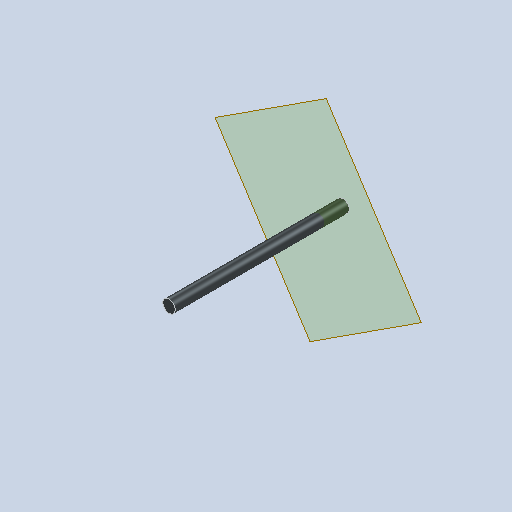
# Autodesk Inventor part: вал
Saved by Autodesk Inventor 2024.2 (Build 282272000, 272)
## iProperties
Created: 2025-11-23
Part Number: вал
Material: Типовые
Document SubType Name: Modeling
Designer: katya_notebook
Density: 1 g/cm^3
Appearance: Чугун серый
Mass: 1.37445 g
Surface Area: 11.3883 cm^2
Volume: 1.37445 cm^3
Author: katya_notebook
Autodesk Inventor part; units mm, degrees
ref_plane "YZ Plane" through (0, 0, 0) normal (1, 0, 0) x (0, 1, 0)
ref_plane "XZ Plane" through (0, 0, 0) normal (0, 1, 0) x (-1, 0, 0)
ref_plane "XY Plane" through (0, 0, 0) normal (0, 0, 1) x (1, 0, 0)
ref_plane "РабПлоскость1" through (-52.9067, -3.7518, -3533.7324) normal (0, 0, -1) x (0.8392895, 0.5436848, 0)
sketch "Эскиз1" plane through (-52.9067, -3.7518, -3533.7324) normal (0, 0, -1) x (0.8392895, 0.5436848, 0)
  circle A0 centre (0, -21.9658) radius 2.6 projected
  circle A1 centre (0, -21.9658) radius 2.5
  point P0 (46.4438, 25.6157)
  dimension "d0" = 5
  constraints: 1 centre point, 1 coincident
  measures "d0" diameter of A1
extrude "Выдавливание1" add sketch "Эскиз1" along normal blind 10 and the other way blind 60 contours A1
